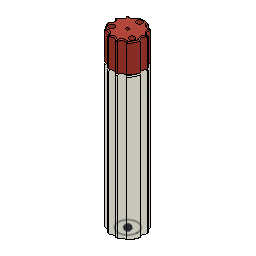
Basket Accu Adapter v5 (Autodesk Fusion 360 design; units mm, degrees)
Autodesk Fusion 360 part; units mm, degrees
note: some values were not read from the file. Set by a fixed rule: which sketch regions a step uses.
sketch "Sketch1" plane through (0, 0, 0) normal (0, 0, 1) x (1, 0, 0)
  line L0 (-9.5, 0) -> (-9.5, 82)
  line L1 (-9.5, 82) -> (-7.5, 82)
  line L2 (-7.5, 82) -> (-7.5, 145)
  line L3 (-7.5, 145) -> (-16.5, 145)
  line L4 (-16.5, 145) -> (-16.5, 0)
  line L5 (-16.5, 0) -> (-9.5, 0)
  line L6 (-16.5, 145) -> (-16.5, 175)
  line L7 (-16.5, 175) -> (0, 175)
  line L8 (0, 175) -> (0, 165)
  line L9 (0, 165) -> (-7.5, 165)
  line L10 (-7.5, 165) -> (-7.5, 145)
  line L11 (-13, 145) -> (-11, 145)
  line L12 (-11, 145) -> (-12, 143.2679)
  line L13 (-12, 143.2679) -> (-13, 145)
  dimension "d1" = 9.5
  dimension "d2" = 16.5
  dimension "d3" = 145
  dimension "d4" = 82
  dimension "d5" = 7.5
  dimension "d6" = 30
  dimension "d7" = 10
  dimension "d8" = 2
  constraint vertical L0
  constraint perpendicular L0 L1
  constraint perpendicular L1 L2
  constraint perpendicular L2 L3
  constraint perpendicular L3 L4
  constraint perpendicular L0 L5
  constraint horizontal origin L0.start
  constraint perpendicular L3 L6
  constraint perpendicular L6 L7
  constraint perpendicular L7 L8
  constraint perpendicular L2 L9
  constraint perpendicular L3 L10
  constraint vertical origin L8.end
  constraint horizontal L11
  constraint equal L11 L12
  constraint equal L11 L13
  constraint midpoint L3 L11
  measures "d1" distance of origin L0
  measures "d2" distance of origin L4
  measures "d3" distance of L3.end L4.end
  measures "d4" distance of L0.start L0.end
  measures "d5" distance of origin L2
  measures "d6" distance of L3.end L6.end
  measures "d7" distance of L7.end L8.end
  measures "d8" distance of L11.start L11.end
revolve "Revolve1" add sketch "Sketch1" angle 360 about axis through (0, 1.75, 0) along (0, 1, 0) contours L0 L1 L2 L3 L4 L5 L12 L13 makes body 1
revolve "Revolve2" add sketch "Sketch1" angle 360 about axis through (0, 1.75, 0) along (0, 1, 0) separate body contours L3 L6 L7 L8 L9 L10 L11 | L3 L11 L12 L13 makes body 2
move_face "OffsetFaces1" offset -0.05 2 faces at (-12.6037, 144.4226, -1.2612) (-11.6087, 143.8453, -1.1616) on bodies 1
chamfer "Chamfer1" distance 1 angle 45 1 edges at (-15.3834, 145, 5.9667) on bodies 1
chamfer "Chamfer2" distance 1 angle 45 1 edges at (-15.3834, 145, 5.9667) on bodies 2
chamfer "Chamfer4" distance 1 angle 45 1 edges at (-15.3834, 0, 5.9667) on bodies 1
chamfer "Chamfer5" distance 3 angle 45 1 edges at (-8.8571, 0, 3.4353) on bodies 1
sketch "Sketch2" plane through (0, 175, 0) normal (0, 1, 0) x (-1, 0, 0)
  circle A0 centre (0, 0) radius 16.5
  point P0 (0, -12)
  dimension "d17" = 12
  constraint vertical A0.centre P0
  measures "d17" vertical distance of A0.centre P0
hole "Hole1" at (0, 175, -12) direction (0, -1, 0) diameter 3.2 end through all counterbore diameter 5.6 counterbore depth 20 bodies 2
pattern_circular "C-Pattern1" count 3 over 360 about axis through (0, 1.75, 0) along (0, 1, 0) of "Hole1"
chamfer "Chamfer6" distance 1 angle 45 1 edges at (-15.3834, 175, 5.9667) on bodies 2
sketch "Sketch3" plane through (0, 165, 0) normal (0, -1, 0) x (1, 0, 0)
  circle A0 centre (0, 0) radius 7.5
  line L0 (2.55, -1.4722) -> (2.55, 1.4722)
  line L1 (2.55, 1.4722) -> (0, 2.9445)
  line L2 (0, 2.9445) -> (-2.55, 1.4722)
  line L3 (-2.55, 1.4722) -> (-2.55, -1.4722)
  line L4 (-2.55, -1.4722) -> (0, -2.9445)
  line L5 (0, -2.9445) -> (2.55, -1.4722)
  dimension "d26" = 2.55
  constraint coincident A0.centre origin
  constraint vertical L4.end A0.centre
  measures "d26" distance of A0.centre L5
extrude "Extrude1" cut sketch "Sketch3" against normal blind 1.5 contours L0 L1 L2 L3 L4 L5 bodies 2
hole "Hole2" at (0, 175, 0) direction (0, -1, 0) diameter 3.1 depth 32.094 tip angle 180 bodies 2
chamfer "Chamfer7" distance 3 angle 45 1 edges at (-6.9925, 165, 2.7121) on bodies 2
hole "Hole4" at (0, 175, -12) direction (0, -1, 0) diameter 2.4 depth 50 tip angle 118 bodies 1
pattern_circular "C-Pattern2" count 3 over 360 about axis through (0, 1.75, 0) along (0, 1, 0) of "Hole4"
sketch "Sketch4" plane through (0, 175, 0) normal (0, 1, 0) x (-1, 0, 0)
  circle A0 centre (0, 0) radius 1.55
  circle A1 centre (-10.3923, 6) radius 2.8
  circle A2 centre (0, -12) radius 2.8
  circle A3 centre (10.3923, 6) radius 2.8
  circle A4 centre (0, 0) radius 15.5
  circle A5 centre (0, -18) radius 4
  circle A6 centre (9, -15.5885) radius 4
  circle A7 centre (15.5885, -9) radius 4
  circle A8 centre (18, 0) radius 4
  circle A9 centre (15.5885, 9) radius 4
  circle A10 centre (9, 15.5885) radius 4
  circle A11 centre (0, 18) radius 4
  circle A12 centre (-9, 15.5885) radius 4
  circle A13 centre (-15.5885, 9) radius 4
  circle A14 centre (-18, 0) radius 4
  circle A15 centre (-15.5885, -9) radius 4
  circle A16 centre (-9, -15.5885) radius 4
  dimension "d41" = 8
  dimension "d42" = 18
  dimension "d44" = 360
  constraint vertical A0.centre A5.centre
  measures "d41" diameter of A5
  measures "d42" distance of A0.centre A5.centre
extrude "Extrude2" cut sketch "Sketch4" against normal up to surface (175 mm away) contours A4 A14 | A4 A14 | A4 A12 | A4 A12 | A4 A15 | A4 A15 | A4 A11 | A4 A11 | A4 A16 | A4 A16 | A4 A10 | A4 A10 | A4 A6 | A4 A6 | A4 A8 | A4 A8 | A4 A7 | A4 A7 bodies 1 2
sketch "Sketch5" plane through (0, 0, 0) normal (0, -1, 0) x (1, 0, 0)
  arc A0 (-10.113, 11.7464) -> (-5.1162, 14.6313) centre (-9, 15.5885) ccw
  arc A1 (-10.113, 11.7464) -> (-15.2292, 2.8849) centre (0, 0) ccw
  arc A2 (-15.2292, -2.8849) -> (-15.2292, 2.8849) centre (-18, 0) ccw
  arc A3 (-15.2292, -2.8849) -> (-14.6313, -5.1162) centre (0, 0) ccw
  arc A4 (-11.7464, -10.113) -> (-14.6313, -5.1162) centre (-15.5885, -9) ccw
  arc A5 (-11.7464, -10.113) -> (-10.113, -11.7464) centre (0, 0) ccw
  arc A6 (-5.1162, -14.6313) -> (-10.113, -11.7464) centre (-9, -15.5885) ccw
  arc A7 (-5.1162, -14.6313) -> (5.1162, -14.6313) centre (0, 0) ccw
  arc A8 (10.113, -11.7464) -> (5.1162, -14.6313) centre (9, -15.5885) ccw
  arc A9 (10.113, -11.7464) -> (11.7464, -10.113) centre (0, 0) ccw
  arc A10 (14.6313, -5.1162) -> (11.7464, -10.113) centre (15.5885, -9) ccw
  arc A11 (14.6313, -5.1162) -> (15.2292, -2.8849) centre (0, 0) ccw
  arc A12 (15.2292, 2.8849) -> (15.2292, -2.8849) centre (18, 0) ccw
  arc A13 (15.2292, 2.8849) -> (10.113, 11.7464) centre (0, 0) ccw
  arc A14 (5.1162, 14.6313) -> (10.113, 11.7464) centre (9, 15.5885) ccw
  arc A15 (5.1162, 14.6313) -> (2.8849, 15.2292) centre (0, 0) ccw
  arc A16 (-2.8849, 15.2292) -> (2.8849, 15.2292) centre (0, 18) ccw
  arc A17 (-2.8849, 15.2292) -> (-5.1162, 14.6313) centre (0, 0) ccw
  circle A18 centre (0, 0) radius 12.5
  circle A19 centre (0, 0) radius 7.5
  circle A20 centre (0, 0) radius 9.5
  point P0 (0, 9.5)
  constraint vertical A1.centre P0
  constraint coincident P0 A20
hole "Hole5" at (0, 0, 9.5) direction (0, 1, 0) diameter 3 depth 82 tip angle 180 bodies 1
pattern_circular "C-Pattern3" count 12 over 360 about axis through (0, 1.75, 0) along (0, 1, 0) of "Hole5"
sketch "Sketch6" plane through (0, 0, 0) normal (0, 1, 0) x (1, 0, 0)
  circle A0 centre (0, 0) radius 9.5
  line L0 (-2.55, -1.4722) -> (0, -2.9445)
  line L1 (0, -2.9445) -> (2.55, -1.4722)
  line L2 (2.55, -1.4722) -> (2.55, 1.4722)
  line L3 (2.55, 1.4722) -> (0, 2.9445)
  line L4 (0, 2.9445) -> (-2.55, 1.4722)
  line L5 (-2.55, 1.4722) -> (-2.55, -1.4722)
  dimension "d52" = 19
  dimension "d53" = 2.55
  constraint coincident A0.centre origin
  constraint vertical A0.centre L0.end
  measures "d52" diameter of A0
  measures "d53" distance of A0.centre L5
extrude "Extrude3" add sketch "Sketch6" along normal blind 10 separate body contours A0 | L0 L1 L2 L3 L4 L5 makes body 3
extrude "Extrude4" cut sketch "Sketch6" along normal blind 1.5 contours L0 L1 L2 L3 L4 L5 bodies 3
hole "Hole6" at (0, 10, 0) direction (0, -1, 0) diameter 3.1 end through all counterbore diameter 5.2 counterbore depth 2 bodies 3
chamfer "Chamfer8" distance 1 angle 45 2 edges at (-8.8571, 10, 3.4353) (-8.8571, 0, 3.4353) on bodies 3
chamfer "Chamfer9" distance 1 angle 45 9 edges at (-7, 175, 12.1244) (0, 175, 14) (7, 175, 12.1244) (14, 175, 0) (12.1244, 175, -7) (7, 175, -12.1244) (-7, 175, -12.1244) (-12.1244, 175, -7) (-14, 175, 0) on bodies 2
equation "d1 = ( 19 / 2 ) * 1 mm"
equation "d2 = ( 33 / 2 ) * 1 mm"
equation "d26 = ( 5.1 / 2 ) * 1 mm"
equation "d53 = ( 5.1 / 2 ) * 1 mm"
named bodies: "Dolni", "Horni", "Vlozka"
